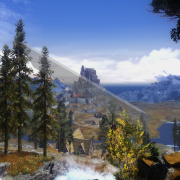
# Autodesk Inventor part: C31_TK_LEDHolder
Saved by Autodesk Inventor 2015 SP1 (Build 190203100, 203)
## iProperties
Created: 2016-02-04
Part Number: C31_TK_LEDHolder
Material: Polycarbonate, Clear
Document SubType Name: Modeling
Designer: TheeTimatahee
Density: 1.2 g/cm^3
Appearance: Polycarbonate - Clear
Author: TheeTimatahee
Autodesk Inventor part; units mm, degrees
ref_plane "YZ Plane" through (0, 0, 0) normal (1, 0, 0) x (0, 1, 0)
ref_plane "XZ Plane" through (0, 0, 0) normal (0, 1, 0) x (-1, 0, 0)
sketch "Sketch1" plane through (0, 0, 0) normal (0, 0, 1) x (1, 0, 0)
  line L0 (-63.5, -8.6463) -> (355.6, -8.6463)
  line L1 (355.6, -8.6463) -> (355.6, 29.4537)
  line L2 (355.6, 29.4537) -> (-63.5, 29.4537)
  line L3 (-63.5, 29.4537) -> (-63.5, -8.6463)
  line L4 (355.6, -8.6463) -> (69.85, -8.6463)
  point P0 (0, 0)
  dimension "d0" = 419.1
  dimension "d27" = 38.1
  constraints: 10 end point, 2 horizontal, 2 parallel, 1 perpendicular, 1 vertical
  measures "d0" distance of L2.end L1.end
  measures "d27" distance of L0.end L1.end
ref_plane "Work Plane1" through (0, 0, 6.35) normal (0, 0, 1) x (1, 0, 0)
sketch "Sketch2" plane through (0, 0, 6.35) normal (0, 0, 1) x (1, 0, 0)
  point P0 (0, 0)
extrude "Extrusion1" add sketch "Sketch1" along normal blind 6.35
fillet "Fillet1" radius 3.175 4 edges at (355.6, 29.4537, 3.175) (355.6, -8.6463, 3.175) (-63.5, 29.4537, 3.175) (-63.5, -8.6463, 3.175)
sketch "Sketch3" plane through (0, 0, 6.35) normal (0, 0, 1) x (1, 0, 0)
  line L0 (-355.6, 35.8037) -> (355.6, 35.8037)
  line L1 (355.6, 35.8037) -> (355.6, 33.2637)
  line L2 (355.6, 33.2637) -> (-355.6, 33.2637)
  line L3 (355.6, -14.9201) -> (-355.6, -14.9201)
  line L4 (355.6, -12.4563) -> (355.6, -14.9201)
  line L5 (355.6, 33.2637) -> (355.6, -12.4563)
  line L6 (-355.6, -12.4563) -> (355.6, -12.4563)
  circle A0 centre (190.5, -2.2201) radius 2.0701
  circle A1 centre (215.9, -2.2201) radius 2.0701
  circle A2 centre (228.6, -2.2201) radius 2.0701
  circle A3 centre (203.2, -2.2201) radius 2.0701
  circle A4 centre (76.2, -2.2963) radius 2.0701
  circle A5 centre (101.6, -2.2963) radius 2.0701
  circle A6 centre (127, -2.2963) radius 2.0701
  circle A7 centre (177.8, -2.2201) radius 2.0701
  constraints: 14 end point, 8 centre point, 6 coincident, 4 horizontal, 3 vertical, 24 other
hole "Hole1" at (76.2, -2.2963, 6.35) at (101.6, -2.2963, 6.35) at (127, -2.2963, 6.35) at (177.8, -2.2201, 6.35) at (203.2, -2.2201, 6.35) at (228.6, -2.2201, 6.35) direction (0, 0, -1) diameter 4.1402 end through all
body "Solid4"
